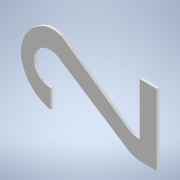
# Autodesk Inventor part: Licence plate numbers
Saved by Autodesk Inventor 2022 (Build 260153070, 153G)
## iProperties
Created: 2021-09-06
Part Number: Licence plate numbers
Material: Generic
Document SubType Name: Modeling
Designer: Main Account
Density: 1 g/cm^3
Appearance: Default
Author: Main Account
Autodesk Inventor part; units mm, degrees
ref_plane "YZ Plane" through (0, 0, 0) normal (1, 0, 0) x (0, 1, 0)
ref_plane "XZ Plane" through (0, 0, 0) normal (0, 1, 0) x (-1, 0, 0)
ref_plane "XY Plane" through (0, 0, 0) normal (0, 0, 1) x (1, 0, 0)
sketch "Sketch1" plane through (0, 0, 0) normal (0, 0, 1) x (1, 0, 0)
  line L0 (-16, -36.75) -> (-16, -53.25) construction
  line L1 (-16, -53.25) -> (16, -53.25) construction
  line L2 (16, -53.25) -> (16, -36.75) construction
  line L3 (16, -36.75) -> (-16, -36.75) construction
  line L4 (-16, -18.75) -> (-16, -35.25) construction
  line L5 (-16, -35.25) -> (16, -35.25) construction
  line L6 (16, -35.25) -> (16, -18.75) construction
  line L7 (16, -18.75) -> (-16, -18.75) construction
  line L8 (-16, -0.75) -> (-16, -17.25) construction
  line L9 (-16, -17.25) -> (16, -17.25) construction
  line L10 (16, -17.25) -> (16, -0.75) construction
  line L11 (16, -0.75) -> (-16, -0.75) construction
  line L12 (-16, 17.25) -> (-16, 0.75) construction
  line L13 (-16, 0.75) -> (16, 0.75) construction
  line L14 (16, 0.75) -> (16, 17.25) construction
  line L15 (16, 17.25) -> (-16, 17.25) construction
  line L16 (-16, 35.25) -> (-16, 18.75) construction
  line L17 (-16, 18.75) -> (16, 18.75) construction
  line L18 (16, 18.75) -> (16, 35.25) construction
  line L19 (16, 35.25) -> (-16, 35.25) construction
  line L20 (-7.7065, -52.162) -> (-7.7065, -48.3518)
  arc A0 (-13.7133, -45.0437) -> (-7.7065, -52.162) centre (-6.1005, -44.7132) ccw
  arc A1 (-8.4582, -38.0516) -> (-13.7133, -45.0437) centre (-6.0975, -45.2967) ccw
  arc A2 (-5.4807, -38.2867) -> (-8.4582, -38.0516) centre (-7.3616, -43.1357) ccw
  line L21 (13.6507, -52.1213) -> (10.7143, -52.1213)
  line L22 (10.2294, -48.3518) -> (10.2294, -37.8422)
  line L23 (10.2294, -37.8422) -> (13.6507, -37.8422)
  line L24 (13.6507, -37.8422) -> (13.6507, -52.1213)
  arc A3 (7.9954, -51.4127) -> (10.7143, -52.1213) centre (10.7143, -46.5506) ccw
  arc A4 (-10.9667, -45.9255) -> (-7.7065, -48.3518) centre (-7.7893, -45.0596) ccw
  arc A5 (-7.7065, -41.7673) -> (-10.9667, -44.1936) centre (-7.7827, -45.0685) ccw
  line L25 (-10.9667, -45.9255) -> (-10.9667, -44.1936)
  arc A6 (-6.2464, -42.1456) -> (-7.7065, -41.7673) centre (-7.7827, -45.0685) ccw
  line L26 (-6.2464, -42.1456) -> (7.9954, -51.4127)
  arc A7 (7.6045, -47.4934) -> (10.2294, -48.3518) centre (10.2482, -43.8521) ccw
  line L27 (7.6045, -47.4934) -> (-5.4807, -38.2867)
  point P0 (0, 0)
  dimension "d6" = 7.62
  dimension "d8" = 7.62
  dimension "d11" = 4.064
  dimension "d12" = 4.064
  dimension "d13" = 3.302
  constraints: 17 point on circle, 16 end point, 8 centre point, 2 parallel, 2 vertical, 1 concentric, 1 horizontal, 1 perpendicular, 1 tangent
  measures "d6" radius of A0
  measures "d8" radius of A1
  measures "d11" distance of L20.end L25.start
  measures "d12" distance of A5.start L25.end
  measures "d13" radius of A5
extrude "Extrusion1" add sketch "Sketch1" along normal blind 0.508
body "Solid1"
